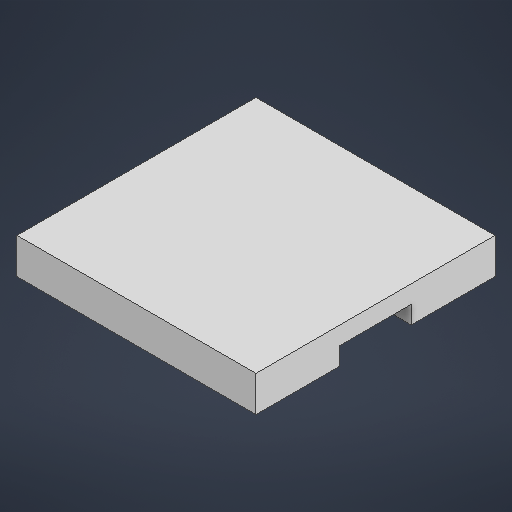
# Autodesk Inventor part: Camera_Housing_Top
Saved by Autodesk Inventor 2026.2 (Build 302298010, 298A)
## iProperties
Created: 2026-02-28
Part Number: Camera_Housing_Top
Material: Generic
Document SubType Name: Modeling
Designer: August
Density: 1 g/cm^3
Appearance: Default
Author: August
Autodesk Inventor part; units mm, degrees
ref_plane "YZ Plane" through (0, 0, 0) normal (1, 0, 0) x (0, 1, 0)
ref_plane "XZ Plane" through (0, 0, 0) normal (0, 1, 0) x (-1, 0, 0)
ref_plane "XY Plane" through (0, 0, 0) normal (0, 0, 1) x (1, 0, 0)
sketch "Sketch1" plane through (0, 0, 0) normal (0, 1, 0) x (-1, 0, 0)
  line L0 (6.7, 6.7) -> (-6.7, 6.7)
  line L1 (-6.7, 6.7) -> (-6.7, -6.7)
  line L2 (-6.7, -6.7) -> (6.7, -6.7)
  line L3 (6.7, -6.7) -> (6.7, 6.7)
  point P0 (0, 0)
  dimension "d0" = 13.4
  dimension "d1" = 13.4
  dimension "d2" = 6.7
  dimension "d3" = 6.7
  constraints: 8 end point, 2 parallel, 1 horizontal, 1 perpendicular
  measures "d0" distance of L2.end L0.start
  measures "d1" distance of L1.end L2.end
  measures "d2" distance from line of point (0, 0) L2
  measures "d3" distance from line of point (0, 0) L3
extrude "Extrusion1" add sketch "Sketch1" along normal blind 2
sketch "Sketch2" plane through (0, 0, 0) normal (0, -1, 0) x (1, 0, 0)
  line L0 (6.7, 6.7) -> (6.7, -6.7) projected
  line L1 (6.7, 6.7) -> (6.7, -6.7)
  line L2 (-6.7, -6.7) -> (-6.7, 6.7) projected
  line L3 (6.7, -6.7) -> (-6.7, -6.7)
  line L4 (-6.7, -6.7) -> (-6.7, 6.7)
  line L5 (-6.7, 6.7) -> (6.7, 6.7)
  line L6 (4.7, 4.7) -> (-4.7, 4.7)
  line L7 (-4.7, 4.7) -> (-4.7, -4.7)
  line L8 (-4.7, -4.7) -> (4.7, -4.7)
  line L9 (4.7, -4.7) -> (4.7, 4.7)
  line L10 (4.7, -2) -> (6.7, -2)
  line L11 (6.7, 2) -> (4.7, 2)
  point P0 (0, 0)
  point P1 (0, 4.7)
  point P2 (5.7, 2)
  point P3 (4.7, 0)
  dimension "d6" = 2
  dimension "d8" = 2
  dimension "d9" = 2
  dimension "d10" = 2
  dimension "d11" = 4
  dimension "d12" = 2
  constraints: 20 end point, 7 perpendicular, 4 point on line, 3 midpoint, 2 collinear, 1 horizontal
  measures "d6" distance between parallel lines of L9 L0
  measures "d8" distance from line of L5 point (0, 4.7)
  measures "d9" distance between parallel lines of L3 L8
  measures "d10" distance between parallel lines of L2 L7
  measures "d11" distance from line of point (5.7, 2) L10
  measures "d12" distance from line of L10 point (4.7, 0)
extrude "Extrusion2" cut sketch "Sketch2" against normal blind 2 contours L0 L10 L9 L11
sketch "Sketch3" plane through (0, 0, 0) normal (0, -1, 0) x (1, 0, 0)
  line L0 (-6.7, -6.7) -> (-6.7, 6.7) projected
  line L1 (-6.7, 2) -> (-4.7, 2)
  line L2 (-4.7, 2) -> (-4.7, -2)
  line L3 (-4.7, -2) -> (-6.7, -2)
  point P0 (0, 0)
  point P1 (-6.7, 0)
  dimension "d15" = 2
  dimension "d16" = 2
  dimension "d17" = 4
  constraints: 6 end point, 2 perpendicular, 2 point on line, 1 horizontal, 1 midpoint
  measures "d15" distance of L1.start L1.end
  measures "d16" distance from line of point (-6.7, 0) L1
  measures "d17" distance of L1.end L2.end
extrude "Extrusion3" cut sketch "Sketch3" against normal blind 1
sketch "Sketch4" plane through (4.7, 0, 2) normal (1, 0, 0) x (0, 0, -1)
  line L0 (0, 2) -> (4, 2) projected
  line L1 (4, 0) -> (4, 1) projected
  line L2 (0, 2) -> (4, 2)
  line L3 (4, 2) -> (4, 1)
  line L4 (4, 1) -> (0, 1)
  line L5 (0, 1) -> (0, 2)
  point P0 (2, 0)
  constraints: 8 end point, 2 parallel, 1 horizontal, 1 perpendicular
extrude "Extrusion4" add sketch "Sketch4" along normal blind 2
sketch "Sketch5" plane through (0, 0, 0) normal (0, -1, 0) x (1, 0, 0)
  line L0 (6.7, 6.7) -> (6.7, 2) projected
  line L1 (-6.7, 2) -> (-6.7, 6.7) projected
  line L2 (6.7, 2.15) -> (-6.7, 2.15)
  line L3 (-6.7, 2.15) -> (-6.7, -2.15)
  line L4 (-6.7, -2.15) -> (6.7, -2.15)
  line L5 (6.7, -2.15) -> (6.7, 2.15)
  line L6 (-4.7, -2) -> (-6.7, -2) projected
  point P0 (0, 0)
  point P1 (-6.7, 2.15)
  dimension "d22" = 4.3
  dimension "d23" = 0.15
  constraints: 8 end point, 2 parallel, 1 horizontal, 1 perpendicular, 1 point on line
  measures "d22" distance of L2.end L3.end
  measures "d23" distance between parallel lines of L6 L4
extrude "Extrusion5" cut sketch "Sketch5" against normal blind 1
sketch "Sketch6" plane through (0, 1, 0) normal (0, -1, 0) x (1, 0, 0)
  line L0 (6.7, 6.7) -> (6.7, -6.7) projected
  line L1 (-6.7, 2) -> (6.7, 2)
  line L2 (6.7, 2) -> (6.7, -2)
  line L3 (6.7, -2) -> (-6.7, -2)
  line L4 (-6.7, -2) -> (-6.7, 2)
  line L5 (-6.7, 2.15) -> (6.7, 2.15) projected
  line L6 (6.7, -2.15) -> (-6.7, -2.15) projected
  line L7 (6.7, -2) -> (6.7, -2.15)
  line L8 (6.7, -2.15) -> (-6.7, -2.15)
  line L9 (-6.7, -2) -> (-6.7, -2.15)
  line L10 (-6.7, 2) -> (-6.7, 2.15)
  line L11 (-6.7, 2.15) -> (6.7, 2.15)
  line L12 (6.7, 2.15) -> (6.7, 2)
  point P0 (0, 0)
  dimension "d26" = 0.15
  dimension "d27" = 0.15
  dimension "d28" = 13.4
  constraints: 20 end point, 3 parallel, 2 collinear, 2 perpendicular, 1 horizontal, 1 point on line
  measures "d26" distance between parallel lines of L5 L1
  measures "d27" distance between parallel lines of L6 L3
  measures "d28" distance between parallel lines of L0 L4
extrude "Extrusion6" add sketch "Sketch6" along normal blind 1 contours L0 L1 L10 L5 | L0 L6 L9 L3
body "Solid1"
